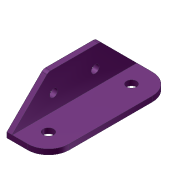
# Autodesk Inventor part: BearingMountBracket
Saved by Autodesk Inventor 2012 (Build 160160000, 160)
## iProperties
Created: 2012-01-26
Part Number: BearingMountBracket
Material: Aluminum-6061
Document SubType Name: Modeling
Designer: JesseK
Density: 2.71 g/cm^3
Mass: 25.5236 g
Surface Area: 68.2319 cm^2
Volume: 9.41831 cm^3
Author: JesseK
Autodesk Inventor part; units mm, degrees
ref_plane "YZ Plane" through (0, 0, 0) normal (1, 0, 0) x (0, 1, 0)
ref_plane "XZ Plane" through (0, 0, 0) normal (0, 1, 0) x (-1, 0, 0)
ref_plane "XY Plane" through (0, 0, 0) normal (0, 0, 1) x (1, 0, 0)
sketch "Sketch1" plane through (0, 0, 0) normal (0, 0, 1) x (1, 0, 0)
  line L0 (0, 0) -> (0, 25.4)
  line L1 (0, 25.4) -> (3.175, 25.4)
  line L2 (3.175, 25.4) -> (3.175, 3.175)
  line L3 (3.175, 3.175) -> (25.4, 3.175)
  line L4 (25.4, 3.175) -> (25.4, 0)
  line L5 (25.4, 0) -> (0, 0)
  dimension "d0" = 3.175
  dimension "d1" = 25.4
  constraints: 12 end point, 3 horizontal, 3 vertical, 2 perpendicular
  measures "d0" distance between parallel lines of L0 L2
  measures "d1" distance of L4.end L0.start
extrude "Extrusion1" add sketch "Sketch1" along normal blind 76.2
sketch "Sketch2" plane through (0, 0, 0) normal (-1, 0, 0) x (0, 0, 1)
  line L0 (76.2, 0) -> (76.2, 25.4) projected
  line L1 (0, 0) -> (0, 25.4) projected
  line L2 (0, 12.7) -> (25.4, 12.7) construction
  line L3 (25.4, 12.7) -> (50.8, 12.7) construction
  line L4 (50.8, 12.7) -> (76.2, 12.7) construction
  circle A0 centre (25.4, 12.7) radius 2.4384
  circle A1 centre (50.8, 12.7) radius 2.4384
  dimension "d4" = 25.4
  dimension "d5" = 4.8768
  constraints: 6 end point, 2 centre point, 2 coincident, 2 horizontal, 2 midpoint, 1 collinear, 1 equal radius
  measures "d4" distance of L2.end L3.end
  measures "d5" diameter of A1
extrude "Extrusion2" cut sketch "Sketch2" against normal up to next
sketch "Sketch3" plane through (0, 0, 0) normal (0, -1, 0) x (1, 0, 0)
  line L0 (25.4, 76.2) -> (0, 76.2) projected
  line L1 (25.4, 0) -> (0, 0) projected
  line L2 (12.7, 76.2) -> (12.7, 63.5) construction
  line L3 (12.7, 63.5) -> (12.7, 12.7) construction
  line L4 (12.7, 12.7) -> (12.7, 0) construction
  circle A0 centre (12.7, 63.5) radius 3.175
  circle A1 centre (12.7, 12.7) radius 3.0898
  dimension "d8" = 6.35
  dimension "d9" = 12.7
  constraints: 6 end point, 2 centre point, 2 coincident, 2 midpoint, 2 vertical, 1 collinear
  measures "d8" diameter of A0
  measures "d9" distance of L3.end L4.end
extrude "Extrusion3" cut sketch "Sketch3" against normal up to next
chamfer "Chamfer1" distance 22.225 angle 45 2 edges at (1.5875, 25.4, 76.2) (1.5875, 25.4, 0)
fillet "Fillet1" radius 12.7 2 edges at (25.4, 1.5875, 76.2) (25.4, 1.5875, 0)
fillet "Fillet2" radius 3.175 2 edges at (1.5875, 25.4, 53.975) (1.5875, 25.4, 22.225)
body "Solid1"
